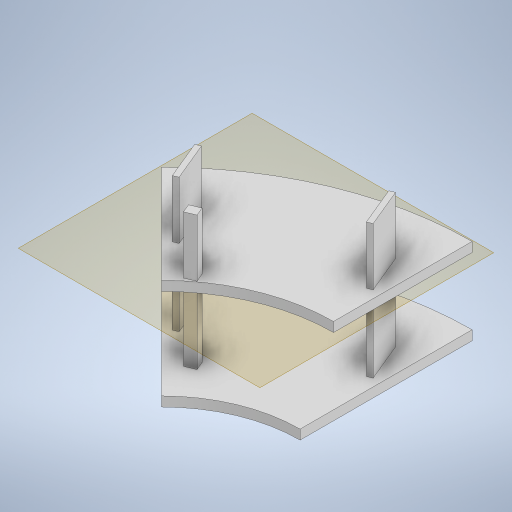
# Autodesk Inventor part: Carousel Container Plate
Saved by Autodesk Inventor 2023 (Build 270158000, 158)
## iProperties
Created: 2022-11-11
Part Number: Carousel Container Plate
Material: Generic
Document SubType Name: Modeling
Designer: cheng
Density: 1 g/cm^3
Appearance: Default
Author: cheng
Autodesk Inventor part; units mm, degrees
ref_plane "YZ Plane" through (0, 0, 0) normal (1, 0, 0) x (0, 1, 0)
ref_plane "XZ Plane" through (0, 0, 0) normal (0, 1, 0) x (-1, 0, 0)
ref_plane "XY Plane" through (0, 0, 0) normal (0, 0, 1) x (1, 0, 0)
sketch "Sketch1" plane through (0, 0, 0) normal (0, 1, 0) x (-1, 0, 0)
  circle A0 centre (0, 0) radius 145
  circle A1 centre (0, 0) radius 325
  line L0 (0, 0) -> (325, 0)
  line L1 (0, 0) -> (0, -325)
  line L2 (0, 0) -> (229.8097, -229.8097)
  line L3 (229.8097, -229.8097) -> (0, -145) construction
  line L4 (1.3869, -199.3328) -> (139.9689, -141.9303)
  line L5 (139.9689, -141.9303) -> (178.2372, -234.3183)
  line L6 (178.2372, -234.3183) -> (39.6553, -291.7208)
  line L7 (39.6553, -291.7208) -> (1.3869, -199.3328)
  line L8 (102.5305, -102.5305) -> (0, -325) construction
  circle A2 centre (0, 0) radius 306.4883 construction
  line L9 (178.2372, -234.3183) -> (1.3869, -199.3328) construction
  line L10 (139.9689, -141.9303) -> (39.6553, -291.7208) construction
  line L11 (89.8121, -216.8255) -> (108.9463, -263.0195) construction
  line L12 (0, 0) -> (124.3721, -300.2608) construction
  line L13 (199.3328, -1.3869) -> (291.7208, -39.6553)
  line L14 (141.9303, -139.9689) -> (199.3328, -1.3869)
  line L15 (234.3183, -178.2372) -> (141.9303, -139.9689)
  line L16 (291.7208, -39.6553) -> (234.3183, -178.2372)
  line L17 (141.9303, 139.9689) -> (234.3183, 178.2372)
  line L18 (199.3328, 1.3869) -> (141.9303, 139.9689)
  line L19 (291.7208, 39.6553) -> (199.3328, 1.3869)
  line L20 (234.3183, 178.2372) -> (291.7208, 39.6553)
  line L21 (1.3869, 199.3328) -> (39.6553, 291.7208)
  line L22 (139.9689, 141.9303) -> (1.3869, 199.3328)
  line L23 (178.2372, 234.3183) -> (139.9689, 141.9303)
  line L24 (39.6553, 291.7208) -> (178.2372, 234.3183)
  line L25 (-139.9689, 141.9303) -> (-178.2372, 234.3183)
  line L26 (-1.3869, 199.3328) -> (-139.9689, 141.9303)
  line L27 (-39.6553, 291.7208) -> (-1.3869, 199.3328)
  line L28 (-178.2372, 234.3183) -> (-39.6553, 291.7208)
  line L29 (-199.3328, 1.3869) -> (-291.7208, 39.6553)
  line L30 (-141.9303, 139.9689) -> (-199.3328, 1.3869)
  line L31 (-234.3183, 178.2372) -> (-141.9303, 139.9689)
  line L32 (-291.7208, 39.6553) -> (-234.3183, 178.2372)
  line L33 (-141.9303, -139.9689) -> (-234.3183, -178.2372)
  line L34 (-199.3328, -1.3869) -> (-141.9303, -139.9689)
  line L35 (-291.7208, -39.6553) -> (-199.3328, -1.3869)
  line L36 (-234.3183, -178.2372) -> (-291.7208, -39.6553)
  line L37 (-1.3869, -199.3328) -> (-39.6553, -291.7208)
  line L38 (-139.9689, -141.9303) -> (-1.3869, -199.3328)
  line L39 (-178.2372, -234.3183) -> (-139.9689, -141.9303)
  line L40 (-39.6553, -291.7208) -> (-178.2372, -234.3183)
  circle A3 centre (0, 0) radius 235 construction
  point P0 (263.0195, -108.9463)
  point P1 (263.0195, 108.9463)
  point P2 (108.9463, 263.0195)
  point P3 (-108.9463, 263.0195)
  point P4 (-263.0195, 108.9463)
  point P5 (-263.0195, -108.9463)
  point P6 (-108.9463, -263.0195)
  dimension "d1" = 180
  dimension "d3" = 45
  dimension "d4" = 650
  dimension "d11" = 150
  dimension "d12" = 100
  dimension "d13" = 22.5
  dimension "d16" = 360
  dimension "d18" = 90
  constraints: 82 end point, 7 point on circle, 4 centre point, 4 coincident, 2 midpoint, 2 parallel, 2 perpendicular, 2 point on line, 1 collinear, 1 horizontal, 73 other
  measures "d1" radial gap between concentric circles of A0 A1
  measures "d3" angle of L1 L2
  measures "d4" diameter of A1
  measures "d11" distance of L5.end L6.end
  measures "d12" distance of L6.end L4.start
  measures "d13" angle of L2 L12
  measures "d18" radial gap between concentric circles of A1 A3
extrude "Extrusion1" add sketch "Sketch1" along normal blind 10 contours A0 L2 A1 L1 | L4 L5 L6 L7
sketch "Sketch2" plane through (0, 10, 0) normal (0, 1, 0) x (1, 0, 0)
  circle A0 centre (0, 0) radius 325
  circle A1 centre (0, 0) radius 145
  line L0 (0, 0) -> (-325, 0)
  line L1 (0, 145) -> (0, 325) projected
  line L2 (0, 0) -> (0, 325)
  arc A2 (0, 325) -> (-229.8097, 229.8097) centre (0, 0) ccw projected
  line L3 (0, 0) -> (-229.8097, 229.8097)
  circle A3 centre (0, 0) radius 235 construction
  line L4 (0, 0) -> (-124.3721, 300.2608) construction
  line L5 (-1.5055, 199.619) -> (-140.0874, 142.2165)
  line L6 (-140.0874, 142.2165) -> (-178.3557, 234.6044)
  line L7 (-178.3557, 234.6044) -> (-39.7738, 292.0069)
  line L8 (-39.7738, 292.0069) -> (-1.5055, 199.619)
  line L9 (-1.5055, 199.619) -> (-178.3557, 234.6044) construction
  line L10 (-140.0874, 142.2165) -> (-39.7738, 292.0069) construction
  circle A4 centre (0, 0) radius 185
  line L11 (-199.619, 1.5055) -> (-292.0069, 39.7738)
  line L12 (-142.2165, 140.0874) -> (-199.619, 1.5055)
  line L13 (-234.6044, 178.3557) -> (-142.2165, 140.0874)
  line L14 (-292.0069, 39.7738) -> (-234.6044, 178.3557)
  line L15 (-199.619, 1.5055) -> (-234.6044, 178.3557) construction
  line L16 (-142.2165, 140.0874) -> (-292.0069, 39.7738) construction
  line L17 (-142.2165, -140.0874) -> (-234.6044, -178.3557)
  line L18 (-199.619, -1.5055) -> (-142.2165, -140.0874)
  line L19 (-292.0069, -39.7738) -> (-199.619, -1.5055)
  line L20 (-234.6044, -178.3557) -> (-292.0069, -39.7738)
  line L21 (-142.2165, -140.0874) -> (-292.0069, -39.7738) construction
  line L22 (-199.619, -1.5055) -> (-234.6044, -178.3557) construction
  line L23 (-1.5055, -199.619) -> (-39.7738, -292.0069)
  line L24 (-140.0874, -142.2165) -> (-1.5055, -199.619)
  line L25 (-178.3557, -234.6044) -> (-140.0874, -142.2165)
  line L26 (-39.7738, -292.0069) -> (-178.3557, -234.6044)
  line L27 (-1.5055, -199.619) -> (-178.3557, -234.6044) construction
  line L28 (-140.0874, -142.2165) -> (-39.7738, -292.0069) construction
  line L29 (140.0874, -142.2165) -> (178.3557, -234.6044)
  line L30 (1.5055, -199.619) -> (140.0874, -142.2165)
  line L31 (39.7738, -292.0069) -> (1.5055, -199.619)
  line L32 (178.3557, -234.6044) -> (39.7738, -292.0069)
  line L33 (140.0874, -142.2165) -> (39.7738, -292.0069) construction
  line L34 (1.5055, -199.619) -> (178.3557, -234.6044) construction
  line L35 (199.619, -1.5055) -> (292.0069, -39.7738)
  line L36 (142.2165, -140.0874) -> (199.619, -1.5055)
  line L37 (234.6044, -178.3557) -> (142.2165, -140.0874)
  line L38 (292.0069, -39.7738) -> (234.6044, -178.3557)
  line L39 (199.619, -1.5055) -> (234.6044, -178.3557) construction
  line L40 (142.2165, -140.0874) -> (292.0069, -39.7738) construction
  line L41 (142.2165, 140.0874) -> (234.6044, 178.3557)
  line L42 (199.619, 1.5055) -> (142.2165, 140.0874)
  line L43 (292.0069, 39.7738) -> (199.619, 1.5055)
  line L44 (234.6044, 178.3557) -> (292.0069, 39.7738)
  line L45 (142.2165, 140.0874) -> (292.0069, 39.7738) construction
  line L46 (199.619, 1.5055) -> (234.6044, 178.3557) construction
  line L47 (1.5055, 199.619) -> (39.7738, 292.0069)
  line L48 (140.0874, 142.2165) -> (1.5055, 199.619)
  line L49 (178.3557, 234.6044) -> (140.0874, 142.2165)
  line L50 (39.7738, 292.0069) -> (178.3557, 234.6044)
  line L51 (1.5055, 199.619) -> (178.3557, 234.6044) construction
  line L52 (140.0874, 142.2165) -> (39.7738, 292.0069) construction
  line L53 (-151.5679, 169.9328) -> (-156.5679, 167.8618)
  line L54 (-156.5679, 167.8618) -> (-173.1364, 207.8618)
  line L55 (-173.1364, 207.8618) -> (-168.1364, 209.9328)
  line L56 (-168.1364, 209.9328) -> (-151.5679, 169.9328)
  line L57 (-151.5679, 169.9328) -> (-173.1364, 207.8618) construction
  line L58 (-156.5679, 167.8618) -> (-168.1364, 209.9328) construction
  line L59 (-12.986, 227.3354) -> (-7.986, 229.4064)
  line L60 (-7.986, 229.4064) -> (-24.5545, 269.4064)
  line L61 (-24.5545, 269.4064) -> (-29.5545, 267.3354)
  line L62 (-12.986, 227.3354) -> (-24.5545, 269.4064) construction
  line L63 (-7.986, 229.4064) -> (-29.5545, 267.3354) construction
  line L64 (-111.6098, 154.0123) -> (-121.6098, 149.8701)
  line L65 (-121.6098, 149.8701) -> (-117.8819, 140.8701)
  line L66 (-117.8819, 140.8701) -> (-107.8819, 145.0123)
  line L67 (-107.8819, 145.0123) -> (-111.6098, 154.0123)
  line L68 (-111.6098, 154.0123) -> (-117.8819, 140.8701) construction
  line L69 (-121.6098, 149.8701) -> (-107.8819, 145.0123) construction
  point P0 (-89.9306, 217.1117)
  point P1 (-217.1117, 89.9306)
  point P2 (-217.1117, -89.9306)
  point P3 (-89.9306, -217.1117)
  point P4 (89.9306, -217.1117)
  point P5 (217.1117, -89.9306)
  point P6 (217.1117, 89.9306)
  point P7 (89.9306, 217.1117)
  point P8 (-68.8241, 166.1562)
  point P9 (-29.5545, 267.3354)
  point P10 (-12.986, 227.3354)
  point P11 (-151.5679, 169.9328)
  dimension "d22" = 180
  dimension "d23" = 650
  dimension "d24" = 90
  dimension "d25" = 100
  dimension "d26" = 150
  dimension "d27" = 40
  dimension "d30" = 360
  dimension "d32" = 40
  dimension "d33" = 5
  dimension "d34" = 9
  dimension "d35" = 10
  dimension "d39" = 30
  dimension "d40" = 20
  constraints: 138 end point, 6 parallel, 4 coincident, 4 symmetric about line, 3 centre point, 3 collinear, 3 perpendicular, 2 midpoint, 2 point on circle, 1 horizontal, 1 point on line, 1 tangent, 1 vertical alignment, 90 other
  measures "d23" diameter of A0
  measures "d24" radial gap between concentric circles of A0 A3
  measures "d25" distance of L7.end L5.start
  measures "d26" distance of L5.start L5.end
  measures "d32" vertical distance of L53.end L54.end
  measures "d33" horizontal distance of L54.end L55.end
  measures "d34" vertical distance of L64.end L65.end
  measures "d35" horizontal distance of L65.end L66.end
  measures "d39" distance between parallel lines of L5 L53
  measures "d40" distance between parallel lines of L6 L65
extrude "Extrusion2" add sketch "Sketch2" along normal blind 140 contours L65 L5 L67 A4 | A4 L67 L66 L65 | L8 L61 L60 L59 | L53 L54 L55 L6
ref_plane "Work Plane1" through (0, 80, 0) normal (0, 1, 0) x (1, 0, 0)
sketch "Sketch4" plane through (0, 80, 0) normal (0, 1, 0) x (1, 0, 0)
  line L0 (-24.5545, 269.4064) -> (-7.986, 229.4064) projected
  line L1 (-7.986, 229.4064) -> (-12.986, 227.3354) projected
  line L2 (-12.986, 227.3354) -> (-29.5545, 267.3354) projected
  line L3 (-29.5545, 267.3354) -> (-24.5545, 269.4064) projected
  line L4 (-156.5679, 167.8618) -> (-173.1364, 207.8618) projected
  line L5 (-173.1364, 207.8618) -> (-168.1364, 209.9328) projected
  line L6 (-168.1364, 209.9328) -> (-151.5679, 169.9328) projected
  line L7 (-151.5679, 169.9328) -> (-156.5679, 167.8618) projected
  line L8 (-107.8819, 145.0123) -> (-117.8819, 140.8701) projected
  line L9 (-117.8819, 140.8701) -> (-121.6098, 149.8701) projected
  line L10 (-121.6098, 149.8701) -> (-111.6098, 154.0123) projected
  line L11 (-111.6098, 154.0123) -> (-107.8819, 145.0123) projected
  arc A0 (0, 145) -> (-102.5305, 102.5305) centre (0, 0) ccw projected
  line L12 (0, 145) -> (0, 325) projected
  arc A1 (0, 325) -> (-229.8097, 229.8097) centre (0, 0) ccw projected
  line L13 (-229.8097, 229.8097) -> (-102.5305, 102.5305) projected
  arc A2 (0, 180) -> (-127.2792, 127.2792) centre (0, 0) ccw
  dimension "d44" = 35
  constraints: 2 point on circle, 2 point on line, 1 centre point, 1 coincident
  measures "d44" radial gap between concentric circles of A0 A2
extrude "Extrusion3" add sketch "Sketch4" along normal blind 10 contours A2 L13 A1 L12
body "Solid1"
